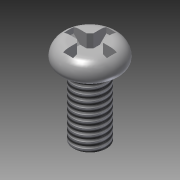
# Autodesk Inventor part: screw_M3_5
Saved by Autodesk Inventor 2013 (Build 170138000, 138)
## iProperties
Shininess: 20.0
Created: 2011-05-14
Part Number: screw_M3_5
Document SubType Name: Modeling
Designer: Noa Izumi
Material: Default
Density: 1 g/cm^3
Density: 0.0
Volumn: 0.0
Area: 0.0
PropertySet Name: Model Information
Control State: 0
Master: False
Checked Out: False
Author: Noa Izumi
Autodesk Inventor part; units mm, degrees
ref_plane "YZ Plane" through (0, 0, 0) normal (1, 0, 0) x (0, 1, 0)
ref_plane "XZ Plane" through (0, 0, 0) normal (0, 1, 0) x (-1, 0, 0)
ref_plane "XY Plane" through (0, 0, 0) normal (0, 0, 1) x (1, 0, 0)
sketch "Sketch1" plane through (0, 0, 0) normal (0, 0, 1) x (1, 0, 0)
  circle A0 centre (0, 0) radius 2.25
  dimension "d0" = 4.5
  constraints: 1 centre point
  measures "d0" diameter of A0
extrude "Extrusion1" add sketch "Sketch1" along normal blind 1.5
fillet "Fillet1" radius 0.5 1 edges at (-2.25, 0, 0)
fillet "Fillet2" radius 1 1 edges at (-2.25, 0, 1.5)
sketch "Sketch2" plane through (0, 0, 1.5) normal (0, 0, 1) x (1, 0, 0)
  line L0 (1.675, 0.375) -> (1.675, -0.375)
  line L1 (-1.625, -0.375) -> (-1.625, 0.375)
  line L2 (-0.375, 1.625) -> (0.375, 1.625)
  line L3 (0.375, -1.675) -> (-0.375, -1.675)
  line L4 (-0.375, -1.675) -> (-0.375, -0.375)
  line L5 (-0.375, 0.375) -> (-0.375, 1.625)
  line L6 (-1.625, 0.375) -> (-0.375, 0.375)
  line L7 (0.375, 0.375) -> (1.675, 0.375)
  line L8 (0.375, 1.625) -> (0.375, 0.375)
  line L9 (0.375, -0.375) -> (0.375, -1.675)
  line L10 (1.675, -0.375) -> (0.375, -0.375)
  line L11 (-0.375, -0.375) -> (-1.625, -0.375)
  circle A0 centre (0, 0) radius 1.25 projected
  dimension "d5" = 0.75
  dimension "d6" = 3.3
  dimension "d9" = 0.75
  dimension "d10" = 3.3
  dimension "d28" = 0.75
  dimension "d29" = 0.75
  dimension "d30" = 0.375
  dimension "d31" = 0.375
  dimension "d32" = 0.375
  dimension "d33" = 0.375
  dimension "d34" = 1.25
  dimension "d35" = 1.25
  constraints: 24 end point, 10 parallel, 4 perpendicular, 3 horizontal
  measures "d5" distance of L1.start L1.end
  measures "d6" distance of L1.end L0.start
  measures "d9" distance of L2.start L2.end
  measures "d10" distance of L2.end L3.start
  measures "d28" distance of L3.start L3.end
  measures "d29" distance of L0.start L0.end
  measures "d30" distance from line of A0.centre L6
  measures "d31" distance from line of A0.centre L7
  measures "d32" distance from line of A0.centre L4
  measures "d33" distance from line of A0.centre L5
  measures "d34" distance between parallel lines of L7 L2
  measures "d35" distance between parallel lines of L5 L1
extrude "Extrusion2" cut sketch "Sketch2" against normal blind 1 contours L0 L10 A0 L7 | A0 L10 L9 L4 L11 L6 L5 L8 L7 | A0 L5 L2 L8 | L9 L3 L4 A0 | A0 L11 L1 L6
chamfer "Chamfer2" distance 0.25 angle 45 4 edges at (-0.375, 0.375, 1) (-0.375, -0.375, 1) (0.375, 0.375, 1) (0.375, -0.375, 1)
sketch "Sketch3" plane through (0, 0, 0) normal (0, 0, -1) x (-1, 0, 0)
  circle A0 centre (0, 0) radius 1.75 projected
  circle A1 centre (0, 0) radius 1.25
  dimension "d19" = 2.5
  constraints: 1 centre point, 1 coincident
  measures "d19" diameter of A1
extrude "Extrusion3" add sketch "Sketch3" along normal blind 5 contours A1
thread "Thread1" size "M2.5x0.45" class "6g" standard "ANSI Metric M Profile" full length
chamfer "倒角3" distance 0.5 angle 45 4 edges at (-1.625, 0, 0.5) (0, 1.625, 0.5) (0, -1.675, 0.5) (1.675, 0, 0.5)
